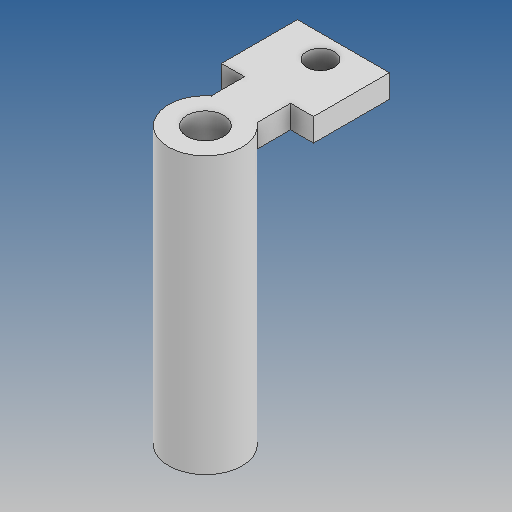
# Autodesk Inventor part: Absicherung Kugellager
Saved by Autodesk Inventor 2026.2 (Build 302298000, 298)
## iProperties
Created: 2026-01-08
Part Number: Absicherung Kugellager
Material: Generisch
Document SubType Name: Modeling
Designer: Schally
Density: 1 g/cm^3
Appearance: Vorgabe
Author: Schally
Autodesk Inventor part; units mm, degrees
ref_plane "YZ Plane" through (0, 0, 0) normal (1, 0, 0) x (0, 1, 0)
ref_plane "XZ Plane" through (0, 0, 0) normal (0, 1, 0) x (-1, 0, 0)
ref_plane "XY Plane" through (0, 0, 0) normal (0, 0, 1) x (1, 0, 0)
sketch "Skizze1" plane through (0, 0, 0) normal (0, 1, 0) x (-1, 0, 0)
  line L0 (10, -8.25) -> (-10, -8.25)
  line L1 (-10, -8.25) -> (-10, 8.25)
  line L2 (-10, 8.25) -> (10, 8.25)
  line L3 (10, 8.25) -> (10, -8.25)
  line L4 (14, 0) -> (-14, 0) projected
  line L5 (0, -16.2) -> (0, 37.7) projected
  circle A0 centre (0, -3.25) radius 3
  line L6 (5, 8.25) -> (-5, 8.25)
  line L7 (-5, 8.25) -> (-5, 16.25)
  line L8 (-5, 16.25) -> (5, 16.25)
  line L9 (5, 16.25) -> (5, 8.25)
  point P0 (0, 0)
  point P1 (-5, 8.25)
  dimension "d0" = 20
  dimension "d1" = 16.5
  dimension "d2" = 6
  dimension "d3" = 11.5
  dimension "d13" = 10
  dimension "d14" = 8
  constraints: 16 end point, 4 parallel, 2 horizontal, 2 perpendicular, 2 point on line, 1 centre point, 3 other
  measures "d0" distance between parallel lines of L1 L3
  measures "d1" distance between parallel lines of L2 L0
  measures "d2" diameter of A0
  measures "d3" distance from line of L2 A0.centre
  measures "d13" distance between parallel lines of L9 L7
  measures "d14" distance between parallel lines of L2 L8
extrude "Extrusion1" add sketch "Skizze1" along normal blind 5 contours L0 L5 A0 L4 L3 | L0 L1 L4 L5 A0 | L4 L5 L2 L3 | L4 L1 L2 L5 | L2 L5 L8 L9 | L2 L7 L8 L5
sketch "Skizze2" plane through (0, 5, 0) normal (0, 1, 0) x (1, 0, 0)
  line L0 (10, -8.25) -> (10, 8.25) projected
  line L1 (10, 8.25) -> (-10, 8.25) projected
  line L2 (-10, 8.25) -> (-10, -8.25) projected
  line L3 (-10, -8.25) -> (-5, -8.25) projected
  circle A0 centre (0, 3.25) radius 3 projected
  line L4 (-2, -8.25) -> (3, -8.25)
  line L5 (-14, 0) -> (14, 0) projected
  line L6 (0, 16.2) -> (0, -37.7) projected
  line L7 (-2.5, -18.25) -> (2.5, -18.25)
  line L8 (2.5, -18.25) -> (2.5, -13.25)
  line L9 (2.5, -13.25) -> (-2.5, -13.25)
  line L10 (-2.5, -13.25) -> (-2.5, -18.25)
  line L11 (-5, -8.25) -> (-5, -16.25) projected
  line L12 (-5, -16.25) -> (5, -16.25) projected
  line L13 (5, -16.25) -> (5, -8.25) projected
  line L14 (5, -8.25) -> (10, -8.25) projected
  circle A1 centre (0, 3.25) radius 3 projected
  circle A2 centre (0, -21.75) radius 4
  circle A3 centre (0, -21.75) radius 8
  line L15 (0, -13.75) -> (0, 3.25)
  point P0 (0, 0)
  dimension "d10" = 5
  dimension "d11" = 5
  dimension "d12" = 5
  dimension "d21" = 8
  dimension "d22" = 25
  dimension "d23" = 4
  constraints: 12 end point, 3 point on line, 2 horizontal, 2 parallel, 1 centre point, 1 collinear, 1 perpendicular, 1 vertical alignment, 3 other
  measures "d10" distance between parallel lines of L7 L9
  measures "d11" distance between parallel lines of L10 L8
  measures "d12" distance between parallel lines of L3 L9
  measures "d21" diameter of A2
  measures "d22" distance of A0.centre A2.centre
  measures "d23" radius of A2
extrude "Extrusion2" add sketch "Skizze2" against normal blind 60 contours A3 L6 A2 L7 L8 L12 L13 | L13 L12 L8 A3 | L8 L12 L6 A3 | L8 L7 A2 L6 L12 | A3 L11 L12 L10 L7 A2 L6 | L6 L12 L10 A3 | L6 A2 L7 L10 L12 | A3 L10 L12 L11
